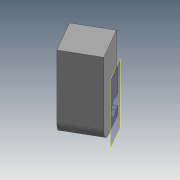
# Autodesk Inventor part: Servo_Mount
Saved by Autodesk Inventor 2014 SP1 (Build 180222100, 222)
## iProperties
Created: 2014-04-09
Part Number: Servo_Mount
Material: Generic
Document SubType Name: Modeling
Designer: tom
Density: 1 g/cm^3
Appearance: Default
Author: tom
Autodesk Inventor part; units mm, degrees
ref_plane "YZ Plane" through (0, 0, 0) normal (1, 0, 0) x (0, 1, 0)
ref_plane "XZ Plane" through (0, 0, 0) normal (0, 1, 0) x (-1, 0, 0)
ref_plane "XY Plane" through (0, 0, 0) normal (0, 0, 1) x (1, 0, 0)
ref_plane "Work Plane1" through (25.296, -13.8947, -14.539) normal (-0.8660254, 0, 0.5) x (0.5, 0, 0.8660254)
sketch "Sketch1" plane through (25.296, -13.8947, -14.539) normal (-0.8660254, 0, 0.5) x (0.5, 0, 0.8660254)
  line L0 (-1.3162, -3.5246) -> (4.1688, -3.5246)
  arc A0 (-0.9285, -1.5996) -> (-0.9285, 1.1504) centre (0.3463, -0.2246) ccw
  line L1 (-0.9285, 1.1504) -> (-2.3162, 1.1504)
  line L2 (-2.3162, -1.5996) -> (-0.9285, -1.5996)
  line L3 (-1.3162, 15.5254) -> (-1.3162, 7.2404)
  line L4 (7.3438, 15.5254) -> (7.3438, -0.3496)
  arc A1 (4.1688, -3.5246) -> (7.3438, -0.3496) centre (4.1688, -0.3496) ccw
  line L5 (-1.3162, 15.5254) -> (7.3438, 15.5254)
  line L6 (-1.6912, 6.8654) -> (-2.3162, 6.8654)
  line L7 (-2.3162, -3.5246) -> (-0.9285, -3.5246)
  line L8 (-2.3162, 6.8654) -> (-2.3162, 1.1504)
  line L9 (-2.3162, -1.5996) -> (-2.3162, -3.5246)
  arc A2 (-1.6912, 6.8654) -> (-1.3162, 7.2404) centre (-1.3162, 6.8654) ccw
  point P0 (-1.3162, -1.5996)
  point P1 (-1.3162, 1.1504)
  dimension "d2" = 3.175
  dimension "d9" = 8.66
  dimension "d10" = 19.05
  dimension "d12" = 15.75
  dimension "d13" = 1.875
  dimension "d14" = 1.375
  dimension "d15" = 1.375
  dimension "d16" = 0.75
  dimension "d17" = 1
  constraints: 20 end point, 6 point on circle, 4 perpendicular, 3 centre point, 3 point on line, 2 tangent, 1 parallel
  measures "d2" radius of A1
  measures "d9" distance between parallel lines of L6 L5
  measures "d10" distance between parallel lines of L0 L5
  measures "d12" distance from line of A0.centre L5
  measures "d13" radius of A0
  measures "d14" distance from line of L1 A0.centre
  measures "d15" distance from line of A0.centre L2
  measures "d16" diameter of A2
  measures "d17" distance from line of L8 A2.centre
extrude "Extrusion1" add sketch "Sketch1" along normal blind 8.66
body "Solid1"
